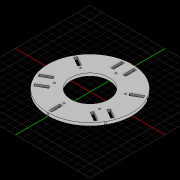
# Autodesk Inventor part: Prototype Plate Base
Saved by Autodesk Inventor 2020.1 (Build 241239000, 239)
## iProperties
Created: 2019-08-27
Part Number: Prototype Plate Base
Material: Generic
Document SubType Name: Modeling
Designer: Oliver Frolovs
Mass: 383.195 g
Surface Area: 1043.06 cm^2
Volume: 383.195 cm^3
Density: 1 g/cm^3
Appearance: Default
Author: Oliver Frolovs
Autodesk Inventor part; units mm, degrees
ref_plane "YZ Plane" through (0, 0, 0) normal (1, 0, 0) x (0, 1, 0)
ref_plane "XZ Plane" through (0, 0, 0) normal (0, 1, 0) x (-1, 0, 0)
ref_plane "XY Plane" through (0, 0, 0) normal (0, 0, 1) x (1, 0, 0)
sketch "Sketch the Prototype Plate Base Profile" plane through (0, 0, 0) normal (0, 0, 1) x (1, 0, 0)
  circle A0 centre (0, 0) radius 135
  dimension "d0" = 270
  constraints: 1 centre point, 1 coincident
  measures "d0" diameter of A0
extrude "Make Prototype Plate Base by Extrusion" add sketch "Sketch the Prototype Plate Base Profile" along normal mid plane 9
sketch "Mark Max Diameter of the Disk" plane through (0, 0, 4.5) normal (0, 0, 1) x (1, 0, 0)
  circle A0 centre (0, 0) radius 61
  dimension "d59" = 122
  constraints: 1 centre point, 1 coincident
  measures "d59" diameter of A0
sketch "Locate the Outer Rib Slots" plane through (0, 0, 4.5) normal (0, 0, 1) x (1, 0, 0)
  circle A0 centre (0, 0) radius 135 projected
  line L0 (0, 0) -> (0, 135) construction
  circle A1 centre (0, 135) radius 15 construction
  line L1 (-24, 125.7578) -> (-15, 125.7578)
  line L2 (-15, 125.7578) -> (-15, 90.7578)
  line L3 (-15, 90.7578) -> (-24, 90.7578)
  line L4 (-24, 90.7578) -> (-24, 125.7578)
  line L5 (-24, 125.7578) -> (-15, 90.7578) construction
  line L6 (-15, 125.7578) -> (-24, 90.7578) construction
  line L7 (-19.5, 108.2578) -> (-15, 108.2578) construction
  circle A2 centre (0, 0) radius 61 construction
  line L8 (24, 125.7578) -> (15, 125.7578)
  line L9 (15, 125.7578) -> (15, 90.7578)
  line L10 (15, 90.7578) -> (24, 90.7578)
  line L11 (24, 90.7578) -> (24, 125.7578)
  circle A3 centre (0, 0) radius 110 construction
  line L12 (-15, 90.7578) -> (0, 90.7578) construction
  dimension "d29" = 220
  dimension "d3" = 30
  dimension "d5" = 35
  dimension "d15" = 9
  dimension "d17" = 122
  dimension "d30" = 15
  constraints: 26 end point, 4 symmetric about line, 3 coincident, 2 centre point, 2 horizontal, 2 midpoint, 2 perpendicular, 1 parallel, 1 point on line, 1 vertical, 1 vertical alignment, 4 other
  measures "d3" diameter of A1
  measures "d5" distance of L3.end L1.start
  measures "d15" distance of L2.end L3.end
  measures "d17" diameter of A2
  measures "d30" distance of L2.end L12.end
extrude "Cut Outer Rib Slots" cut sketch "Locate the Outer Rib Slots" against normal blind 9 contours L1 L2 L3 L4 | L11 L10 L9 L8
pattern_circular "Pattern Outer Rib Slots Around the Base Plate" count 3 over 360 about axis through (0, 0, -10) along (0, 0, 1) of "Cut Outer Rib Slots"
sketch "Locate the Inner Rib Slot" plane through (0, 0, 4.5) normal (0, 0, 1) x (1, 0, 0)
  circle A0 centre (0, 0) radius 135 projected
  line L0 (-112.6682, 59.8529) -> (-108.1682, 67.6471)
  line L1 (-108.1682, 67.6471) -> (-77.8573, 50.1471)
  line L2 (-77.8573, 50.1471) -> (-82.3573, 42.3529)
  line L3 (-82.3573, 42.3529) -> (-112.6682, 59.8529)
  line L4 (-112.6682, 59.8529) -> (-77.8573, 50.1471) construction
  line L5 (-108.1682, 67.6471) -> (-82.3573, 42.3529) construction
  circle A1 centre (0, 0) radius 110 construction
  line L6 (-95.2628, 55) -> (0, 0) construction
  line L7 (0, -210) -> (0, 210) projected
  dimension "d31" = 220
  dimension "d27" = 9
  dimension "d28" = 35
  dimension "d32" = 60
  constraints: 14 end point, 2 midpoint, 2 parallel, 2 perpendicular, 1 coincident, 3 other
  measures "d27" distance of L1.end L2.end
  measures "d28" distance of L0.end L1.end
  measures "d32" angle of L7 L6
extrude "Cut Inner Rib Slots" cut sketch "Locate the Inner Rib Slot" against normal blind 9 contours L0 L1 L2 L3
pattern_circular "Pattern Inner Rib Slots Around the Base Plate" count 3 over 360 about axis through (0, 0, -10) along (0, 0, 1) of "Cut Inner Rib Slots"
sketch "Locate Holes for Connecting Two Bases" plane through (0, 0, 4.5) normal (0, 0, 1) x (1, 0, 0)
  circle A0 centre (0, 0) radius 135 projected
  line L0 (-15, 125.7578) -> (-15, 90.7578) projected
  line L1 (15, 90.7578) -> (15, 125.7578) projected
  line L2 (0, 136.5) -> (0, 83.5) construction
  circle A1 centre (0, 0) radius 110 construction
  point P0 (0, 110)
  point P1 (-118.2125, 68.25)
  point P2 (-72.3131, 41.75)
  point P3 (-118.2125, -68.25)
  point P4 (-72.3131, -41.75)
  point P5 (0, -136.5)
  point P6 (0, -83.5)
  point P7 (118.2125, -68.25)
  point P8 (72.3131, -41.75)
  point P9 (118.2125, 68.25)
  point P10 (72.3131, 41.75)
  dimension "d54" = 220
  dimension "d49" = 53
  dimension "d57" = 360
  constraints: 2 end point, 1 coincident, 1 midpoint, 1 point on line, 1 vertical, 1 vertical alignment, 15 other
  measures "d49" distance of L2.start L2.end
hole "Drill M5 Close Clearance Holes for Connecting Two Bases" at (0, 136.5, 4.5) at (0, 83.5, 4.5) at (118.2125, 68.25, 4.5) at (72.3131, 41.75, 4.5) at (-72.3131, 41.75, 4.5) at (-118.2125, 68.25, 4.5) at (-72.3131, -41.75, 4.5) at (-118.2125, -68.25, 4.5) at (0, -83.5, 4.5) at (0, -136.5, 4.5) at (72.3131, -41.75, 4.5) at (118.2125, -68.25, 4.5) direction (0, 0, -1) diameter 5.3 end through all clearance for "Socket Head Cap Screw ISO 4762" size "M5" standard "ISO"
extrude "Cut Out Centre of the Base Plate to DISK SIZE ONLY" cut sketch "Mark Max Diameter of the Disk" against normal blind 9
equation "\"d0\" = PrototypePlateDiameter"
equation "\"d1\" = PrototypePlateMaterialThickness"
equation "\"d59\" = RigDiskMaxDiameter"
equation "\"d29\" = OuterRibSlotPCD"
equation "\"d3\" = RigColumnsDiameter"
equation "\"d5\" = RibSlotLength"
equation "\"d15\" = PrototypePlateRibMaterialThickness"
equation "\"d30\" = 0.5 * RigColumnsDiameter"
equation "\"d18\" = PrototypePlateMaterialThickness"
equation "\"d31\" = InnerRibSlotPCD"
equation "\"d27\" = PrototypePlateRibMaterialThickness"
equation "\"d28\" = RibSlotLength"
equation "\"d33\" = PrototypePlateMaterialThickness"
equation "\"d54\" = InnerRibSlotPCD"
equation "\"d60\" = PrototypePlateMaterialThickness"
equation "\"PrototypePlateDiameter\" = 270"
equation "\"PrototypePlateMaterialThickness\" = 9"
equation "\"RigDiskMaxDiameter\" = 122"
equation "\"OuterRibSlotPCD\" = 220"
equation "\"RigColumnsDiameter\" = 30"
equation "\"RibSlotLength\" = 35"
equation "\"PrototypePlateRibMaterialThickness\" = 9"
equation "\"InnerRibSlotPCD\" = 220"
body "Solid1"
